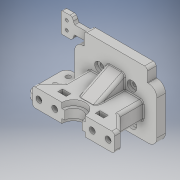
# Autodesk Inventor part: Froggie_DualFan_BLTouchMount01
Saved by Autodesk Inventor 2019.4 (Build 234330000, 330)
## iProperties
Created: 2019-11-18
Part Number: Froggie_DualFan_BLTouchMount01
Material: Generic
Document SubType Name: Modeling
Designer: frogm
Density: 1 g/cm^3
Appearance: Default
Author: frogm
Autodesk Inventor part; units mm, degrees
ref_plane "XZ Plane" through (0, 0, 0) normal (0, 1, 0) x (-1, 0, 0)
ref_plane "XY Plane" through (0, 0, 0) normal (0, 0, 1) x (1, 0, 0)
sketch "Base Sketch" plane through (0, 0, 0) normal (0, 0, 1) x (1, 0, 0)
  line L0 (0, 54) -> (0, -9) construction
  line L1 (-39.9, 0) -> (39.9, 0) construction
  line L2 (-28.5, 0) -> (28.5, 0)
  line L3 (-28.5, 0) -> (-28.5, 36)
  line L4 (-28.5, 36) -> (-22, 36)
  line L5 (-22, 36) -> (-22, 45)
  line L6 (-22, 45) -> (22, 45)
  line L7 (22, 45) -> (22, 36)
  line L8 (22, 36) -> (28.5, 36)
  line L9 (28.5, 36) -> (28.5, 0)
  point P0 (0, 0)
  point P1 (0, 0)
  dimension "d0" = 57
  dimension "d1" = 36
  dimension "d2" = 6.5
  dimension "d3" = 9
  dimension "d4" = 44
  dimension "d5" = 9
  dimension "d6" = 6.5
  dimension "d37" = 36
  constraints: 16 end point, 5 point on line, 4 perpendicular, 1 midpoint
  measures "d0" distance of L2.start L2.end
  measures "d1" distance of L2.start L3.end
  measures "d2" distance of L3.end L4.end
  measures "d3" distance of L4.end L5.end
  measures "d4" distance of L5.end L6.end
  measures "d5" distance of L6.end L7.end
  measures "d6" distance of L7.end L8.end
  measures "d37" distance of L8.end L2.end
extrude "Base Extrusion (6)" add sketch "Base Sketch" along normal blind 6
sketch "Base Holes Sketch" plane through (0, 0, 6) normal (0, 0, 1) x (1, 0, 0)
  line L0 (0, 0) -> (0, 44.9253) construction
  circle A0 centre (-11.25, 6.2) radius 1.5
  line L1 (-28.5, 0) -> (28.5, 0) projected
  circle A1 centre (11.25, 6.2) radius 1.5
  circle A2 centre (-11.25, 28.7) radius 1.5
  circle A3 centre (11.25, 28.7) radius 1.5
  circle A4 centre (-11.25, 6.2) radius 3.325
  circle A5 centre (11.25, 6.2) radius 3.325
  circle A6 centre (11.25, 28.7) radius 3.325
  circle A7 centre (-11.25, 28.7) radius 3.325
  dimension "d9" = 3
  dimension "d10" = 6.2
  dimension "d11" = 11.25
  dimension "d14" = 22.5
  dimension "d19" = 6.65
  dimension "d20" = 6.65
  dimension "d21" = 6.65
  dimension "d22" = 6.65
  constraints: 8 centre point, 4 coincident, 2 end point, 2 vertical, 1 symmetric about line, 5 other
  measures "d9" diameter of A0
  measures "d10" distance from line of L1 A0.centre
  measures "d11" distance from line of L0 A0.centre
  measures "d14" distance of A0.centre A2.centre
  measures "d19" diameter of A4
  measures "d20" diameter of A5
  measures "d21" diameter of A6
  measures "d22" diameter of A7
extrude "Base Screw Holes (Through)" cut sketch "Base Holes Sketch" against normal up to surface (6 mm away) contours A0 | A1 | A2 | A3
extrude "Counterbore Base Screws (2)" cut sketch "Base Holes Sketch" against normal blind 2
sketch "Heatsink Platform Sketch" plane through (0, 0, 6) normal (0, 0, 1) x (1, 0, 0)
  line L0 (28.5, 0) -> (28.5, 36) construction
  line L1 (-28.5, 36) -> (-28.5, 0) construction
  line L2 (-28.5, 17.45) -> (28.5, 17.45) construction
  circle A0 centre (-11.25, 28.7) radius 1.5 construction
  line L3 (-28.5, 23.8) -> (28.5, 23.8)
  line L4 (28.5, 23.8) -> (28.5, 11.1)
  line L5 (28.5, 11.1) -> (-28.5, 11.1)
  line L6 (-28.5, 11.1) -> (-28.5, 23.8)
  point P0 (0, 0)
  dimension "d27" = 11.25
  dimension "d28" = 12.7
  constraints: 10 end point, 5 point on line, 2 parallel, 2 perpendicular, 1 horizontal, 1 midpoint
  measures "d27" distance from line of A0.centre L2
  measures "d28" distance of L3.end L4.end
extrude "Heatsink Platform Extrusion (29.25)" add sketch "Heatsink Platform Sketch" along normal blind 29.25
sketch "Heatsink Platform Cutaway Sketch" plane through (-28.5, 23.8, 6) normal (0, 1, 0) x (1, 0, 0)
  line L0 (57, -29.25) -> (0, -29.25) construction
  line L1 (28.5, -29.25) -> (28.5, 0) construction
  line L2 (57, 0) -> (0, 0) construction
  line L3 (9.5, -16) -> (9.5, 0)
  line L4 (9.5, -16) -> (0, -25.35)
  line L5 (0, -25.35) -> (0, 0)
  line L6 (0, 0) -> (9.5, 0)
  line L7 (47.5, -16) -> (47.5, 0)
  line L8 (47.5, -16) -> (57, -25.35)
  line L9 (57, -25.35) -> (57, 0)
  line L10 (57, 0) -> (47.5, 0)
  point P0 (28.5, 6)
  dimension "d31" = 19
  dimension "d32" = 16
  dimension "d33" = 25.35
  constraints: 18 end point, 3 symmetric about line, 2 midpoint, 1 collinear, 1 perpendicular, 1 point on line
  measures "d31" distance from line of L1 L3.start
  measures "d32" distance from line of L2 L3.start
  measures "d33" distance from line of L2 L4.end
extrude "Heatsink Platform Cutaway Extrusion" cut sketch "Heatsink Platform Cutaway Sketch" against normal up to surface (12.7 mm away)
fillet "Heatsink Platform Trim Fillet (2)" radius 2 12 edges at (28.5, 23.8, 33.3) (23.75, 23.8, 26.675) (19, 23.8, 14) (19, 11.1, 14) (23.75, 11.1, 26.675) (28.5, 11.1, 33.3) (-19, 23.8, 14) (-23.75, 23.8, 26.675) (-28.5, 23.8, 33.3) (-28.5, 11.1, 33.3) (-23.75, 11.1, 26.675) (-19, 11.1, 14)
sketch "Heatsink Extrusion sketch" plane through (-17, 23.8, 6) normal (0, 1, 0) x (1, 0, 0)
  line L0 (43.5, -29.25) -> (-9.5, -29.25) projected
  arc A0 (23, -29.25) -> (11, -29.25) centre (17, -29.25) ccw
  arc A1 (25, -29.25) -> (9, -29.25) centre (17, -29.25) ccw
  line L1 (17, -29.25) -> (9, -29.25) construction
  line L2 (17, -29.25) -> (25, -29.25) construction
  line L3 (9, -29.25) -> (11, -29.25)
  line L4 (23, -29.25) -> (25, -29.25)
  line L5 (11, -29.25) -> (23, -29.25)
  point P0 (17, 6)
  dimension "d38" = 6
  dimension "d39" = 8
  dimension "d40" = 180
  constraints: 10 end point, 4 point on circle, 3 point on line, 2 centre point, 2 coincident, 2 collinear, 1 midpoint
  measures "d38" radius of A0
  measures "d39" radius of A1
  measures "d40" angle of L2 L1
extrude "Heatsink Center Extrusion (6)" cut sketch "Heatsink Extrusion sketch" against normal up to surface (12.7 mm away) contours L0 A0
extrude "Heastsink Top Outer Extrusion (3.7)" cut sketch "Heatsink Extrusion sketch" against normal blind 3.7 contours L0 A0 A1
sketch "Heatsink Bottom Extrusion Sketch" plane through (-17, 11.1, 6) normal (0, -1, 0) x (1, 0, 0)
  line L0 (11, 29.25) -> (9, 29.25) projected
  arc A0 (9, 29.25) -> (25, 29.25) centre (17, 29.25) ccw projected
  line L1 (25, 29.25) -> (23, 29.25) projected
  arc A1 (11, 29.25) -> (23, 29.25) centre (17, 29.25) ccw projected
  point P0 (17, -6)
extrude "Heatsink Bottom Outer Extrusion (3.0)" cut sketch "Heatsink Bottom Extrusion Sketch" against normal blind 3
ref_plane "Front Screw Hole Plane" through (0, 0, 35.25) normal (0, 0, 1) x (1, 0, 0)
sketch "Front Screw Hole Sketch" plane through (0, 0, 35.25) normal (0, 0, 1) x (1, 0, 0)
  line L0 (-8, 23.8) -> (-26.5, 23.8) construction
  line L1 (-8, 17.45) -> (-26.5, 17.45) construction
  line L2 (-28.5, 36) -> (-28.5, 0) construction
  line L3 (-28.5, 17.45) -> (28.5, 17.45) construction
  line L4 (-28.5, 17.45) -> (28.5, 17.45) construction
  line L5 (8, 11.1) -> (-8, 11.1) construction
  line L6 (0, 11.1) -> (0, 23.8) construction
  circle A0 centre (13, 17.45) radius 2.05
  circle A1 centre (-13, 17.45) radius 2.05
  circle A2 centre (24, 17.45) radius 2.05
  line L7 (28.5, 13.1) -> (28.5, 21.8) projected
  circle A3 centre (-24, 17.45) radius 2.05
  point P0 (0, 0)
  dimension "d48" = 6.35
  dimension "d49" = 57
  dimension "d50" = 0
  dimension "d51" = 4.1
  dimension "d52" = 13
  dimension "d53" = 4.1
  dimension "d54" = 4.5
  constraints: 8 end point, 4 centre point, 3 point on line, 2 collinear, 2 symmetric about line, 1 horizontal, 1 midpoint, 1 parallel, 1 vertical, 2 other
  measures "d48" distance between parallel lines of L0 L1
  measures "d49" distance of L3.start L3.end
  measures "d50" distance between parallel lines of L3 L4
  measures "d51" diameter of A0
  measures "d52" distance from line of L6 A0.centre
  measures "d53" diameter of A2
  measures "d54" distance from line of A2.centre L7
extrude "Heatsink Screw Hole Extrusion (14)" cut sketch "Front Screw Hole Sketch" against normal blind 14 contours A0 | A1
extrude "Hotend Cooling Fan Screw Holes Extrusion (To Next)" cut sketch "Front Screw Hole Sketch" against normal up to next contours A2 | A3
sketch "Nut-trap Sketch" plane through (-17, 23.8, 6) normal (0, 1, 0) x (1, 0, 0)
  arc A0 (25, -29.25) -> (9, -29.25) centre (17, -29.25) ccw construction
  line L0 (17, -21.25) -> (17, 0) construction
  line L1 (34, 0) -> (0, 0) construction
  line L2 (1.1, -24.25) -> (6.9, -24.25)
  line L3 (6.9, -24.25) -> (6.9, -21.05)
  line L4 (6.9, -21.05) -> (1.1, -21.05)
  line L5 (1.1, -21.05) -> (1.1, -24.25)
  line L6 (9, -29.25) -> (-9.5, -29.25) projected
  line L7 (32.9, -24.25) -> (27.1, -24.25)
  line L8 (27.1, -24.25) -> (27.1, -21.05)
  line L9 (27.1, -21.05) -> (32.9, -21.05)
  line L10 (32.9, -21.05) -> (32.9, -24.25)
  point P0 (17, 6)
  point P1 (4, -21.05)
  dimension "d59" = 5.8
  dimension "d60" = 3.2
  dimension "d61" = 5
  dimension "d62" = 13
  constraints: 18 end point, 4 symmetric about line, 2 midpoint, 2 parallel, 1 horizontal, 1 perpendicular, 1 point on circle, 1 vertical
  measures "d59" distance of L4.end L3.end
  measures "d60" distance of L3.end L2.end
  measures "d61" distance between parallel lines of L6 L2
  measures "d62" distance from line of L0 point (4, -21.05)
extrude "Nut-trap Extrusion (9.03)" cut sketch "Nut-trap Sketch" against normal blind 9.03
ref_plane "Cooling Fan Nut Sketch Plane" through (-17, 23.8, 22.8378) normal (0, 0, -1) x (-1, 0, 0)
sketch "Cooling Fan Nut Sketch" plane through (-17, 23.8, 22.8378) normal (0, 0, -1) x (-1, 0, 0)
  line L0 (3.8823, -6.3515) -> (5.4425, -9.0508)
  line L1 (5.4425, -9.0508) -> (8.5602, -9.0492)
  line L2 (8.5602, -9.0492) -> (10.1177, -6.3485)
  line L3 (10.1177, -6.3485) -> (8.5575, -3.6492)
  line L4 (8.5575, -3.6492) -> (5.4398, -3.6508)
  line L5 (5.4398, -3.6508) -> (3.8823, -6.3515)
  line L6 (7.0013, -9.05) -> (6.9987, -3.65) construction
  circle A0 centre (7, -6.35) radius 2.05 projected
  line L7 (-25, 0) -> (-9, 0) projected
  line L8 (-17, 0) -> (-17, -12.7) construction
  line L9 (-34, -12.7) -> (0, -12.7) projected
  line L10 (-37.8823, -6.3515) -> (-39.4425, -9.0508)
  line L11 (-39.4425, -9.0508) -> (-42.5602, -9.0492)
  line L12 (-42.5602, -9.0492) -> (-44.1177, -6.3485)
  line L13 (-44.1177, -6.3485) -> (-42.5575, -3.6492)
  line L14 (-42.5575, -3.6492) -> (-39.4398, -3.6508)
  line L15 (-39.4398, -3.6508) -> (-37.8823, -6.3515)
  point P0 (-17, -23.8)
  point P1 (7, -6.35)
  constraints: 28 end point, 6 symmetric about line, 5 midpoint
extrude "Cooling Fan Nut Extrusion (10.25)" cut sketch "Cooling Fan Nut Sketch" against normal blind 10.25 contours L5 L4 L3 L2 L1 L0 | A0 | L10 L11 L12 L13 L14 L15
ref_plane "Support Brace Plane" through (6.3, 0, 0) normal (1, 0, 0) x (0, 1, 0)
sketch "Top Support Brace Sketch" plane through (6.3, 0, 0) normal (1, 0, 0) x (0, 1, 0)
  line L0 (23.8, 6) -> (23.8, 26)
  line L1 (23.8, 6) -> (23.8, 22.8378) projected
  line L2 (23.8, 6) -> (33.8, 6)
  line L3 (33.8, 6) -> (23.8, 26)
  point P0 (0, 0)
  dimension "d68" = 20
  dimension "d69" = 10
  constraints: 6 end point, 1 collinear
  measures "d68" distance of L0.start L0.end
  measures "d69" distance of L0.start L2.end
extrude "Top Support Brace Extrusion (12.6)" add sketch "Top Support Brace Sketch" against normal blind 12.6
fillet "Support Base Trim Fillet (2)" radius 2 2 edges at (6.3, 28.8, 16) (-6.3, 28.8, 16)
fillet "Support Base Congruent Fillet (.6)" radius 0.6 10 edges at (5.7142, 23.8, 24.6901) (0, 23.8, 26) (-5.7142, 23.8, 24.6901) (-6.3, 23.8, 13.7639) (6.3, 23.8, 13.7639) (5.7142, 33.1451, 6) (0, 33.8, 6) (-5.7142, 33.1451, 6) (-6.3, 27.682, 6) (6.3, 27.682, 6)
fillet "Heatsink Platform Congruent Fillet (.6)" radius 0.6 11 edges at (11.95, 23.8, 6) (6.4757, 23.9757, 6.1757) (19, 17.45, 6) (18.4142, 11.6858, 6) (0, 11.1, 6) (-18.4142, 11.6858, 6) (-19, 17.45, 6) (-18.4142, 23.2142, 6) (-11.95, 23.8, 6) (-6.4757, 23.9757, 6.1757) (18.4142, 23.2142, 6)
ref_plane "Support Base Cross Section Plane" through (-17, 17.45, 22.8378) normal (0, 1, 0) x (1, 0, 0)
mirror "Support Base Mirror" about plane through (-17, 17.45, 22.8378) normal (0, 1, 0) of "Top Support Brace Extrusion (12.6)", "Support Base Trim Fillet (2)", "Support Base Congruent Fillet (.6)"
fillet "Base Large Fillet (6)" radius 6 4 edges at (28.5, 0, 3) (28.5, 36, 3) (-28.5, 36, 3) (-28.5, 0, 3)
fillet "Base Small Fillet (3)" radius 2 2 edges at (-22, 45, 3) (22, 45, 3)
ref_plane "BL Touch Platform Plane" through (-22.5, 6.75, 0) normal (0, -1, 0) x (1, 0, 0)
sketch "BL Touch Platform Sketch" plane through (-22.5, 6.75, 0) normal (0, -1, 0) x (1, 0, 0)
  line L0 (-6, 0) -> (-17.6, 0)
  line L1 (-17.6, 0) -> (-17.6, 27.5)
  line L2 (-17.6, 27.5) -> (-6, 27.5)
  line L3 (-6, 27.5) -> (-6, 0)
  point P0 (22.5, 0)
  dimension "d79" = 11.6
  dimension "d80" = 27.5
  constraints: 8 end point, 2 parallel, 1 horizontal, 1 perpendicular
  measures "d79" distance of L1.end L2.end
  measures "d80" distance of L0.end L1.end
extrude "BL Touch Platform Extrusion (4)" add sketch "BL Touch Platform Sketch" against normal blind 4
fillet "BL Touch Platform Trim Fillet (4.5)" radius 4.5 3 edges at (-40.1, 8.75, 0) (-40.1, 8.75, 27.5) (-28.5, 8.75, 27.5)
sketch "BL Touch Platform Holes Sketch" plane through (-22.5, 10.75, 0) normal (0, 1, 0) x (1, 0, 0)
  circle A0 centre (-11.765, -22.73) radius 1.6
  circle A1 centre (-11.765, -13.73) radius 1.6
  circle A2 centre (-11.765, -4.73) radius 1.6
  point P0 (22.5, 0)
  point P1 (22.5, -4)
  dimension "d86" = 3.2
  dimension "d91" = 3.2
  constraints: 3 centre point, 1 coincident
  measures "d86" diameter of A2
  measures "d91" diameter of A1
extrude "BL Touch Screw Holes Extrusion (Through)" cut sketch "BL Touch Platform Holes Sketch" against normal up to surface (4 mm away)
sketch "Endstop Holder Sketch" plane through (0, 0, 0) normal (0, 0, 1) x (1, 0, 0)
  line L0 (-31.8142, 34.5) -> (-31.8142, 32.7426) construction
  line L1 (-34.764, 32.3787) -> (-39.9355, 32.3787)
  arc A0 (-34.764, 32.3787) -> (-33.3497, 32.9645) centre (-34.764, 34.3787) ccw
  arc A1 (-40.9355, 33.3787) -> (-39.9355, 32.3787) centre (-39.9355, 33.3787) ccw
  arc A2 (-33.3497, 46.0355) -> (-34.764, 46.6213) centre (-34.764, 44.6213) ccw
  line L2 (-34.764, 46.6213) -> (-39.9355, 46.6213)
  arc A3 (-39.9355, 46.6213) -> (-40.9355, 45.6213) centre (-39.9355, 45.6213) ccw
  line L3 (-40.9355, 33.3787) -> (-40.9355, 45.6213)
  line L4 (-36.9355, 32.3787) -> (-36.9355, 46.6213) construction
  circle A4 centre (-36.9355, 36.5002) radius 1
  circle A5 centre (-36.9355, 42.5002) radius 1
  line L5 (-40.9355, 39.5) -> (-24.6363, 39.5) construction
  arc A6 (-32.2633, 44.3544) -> (-31.4, 42.5) centre (-28.7972, 44.8399) ccw
  arc A7 (-32.2633, 44.3544) -> (-33.3497, 46.0355) centre (-36.2903, 42.9436) ccw
  arc A8 (-31.4, 36.5) -> (-32.2633, 34.6456) centre (-28.7972, 34.1601) ccw
  arc A9 (-33.3497, 32.9645) -> (-32.2633, 34.6456) centre (-36.2903, 36.0564) ccw
  line L6 (-31.4, 42.5) -> (-22, 42.5)
  line L7 (-31.4, 36.5) -> (-22, 36.5)
  line L8 (-22, 36.5) -> (-22, 42.5)
  point P0 (-33.9355, 32.3787)
  point P1 (-40.9355, 32.3787)
  point P2 (-40.9355, 47.3787)
  point P3 (-33.9355, 47.3787)
  point P4 (-22, 36)
  dimension "d97" = 3
  dimension "d99" = 7
  dimension "d100" = 15
  dimension "d101" = 7
  dimension "d102" = 1
  dimension "d106" = 4
  dimension "d107" = 4.1215
  dimension "d108" = 6
  dimension "d109" = 4.1211
  dimension "d110" = 2
  dimension "d111" = 2
  dimension "d117" = 3.5
  dimension "d119" = 9.4
  constraints: 18 end point, 16 point on circle, 10 centre point, 4 point on line, 3 horizontal, 2 coincident, 2 tangent, 1 perpendicular
  measures "d97" distance of L0.start point (-33.936, 32.379)
  measures "d99" distance of point (-33.936, 32.379) point (-40.936, 32.379)
  measures "d100" distance of point (-40.936, 32.379) point (-40.936, 47.379)
  measures "d101" distance of point (-40.936, 47.379) point (-33.936, 47.379)
  measures "d102" radius of A1
  measures "d106" distance between parallel lines of L3 L4
  measures "d107" distance from line of L1 point (-36.936, 36.5)
  measures "d108" distance of point (-36.936, 36.5) point (-36.936, 42.5)
  measures "d109" distance from line of point (-36.936, 42.5) L2
  measures "d110" diameter of A4
  measures "d111" diameter of A5
  measures "d117" radius of A6
  measures "d119" distance of L6.start L6.end
extrude "Endstop Holder Extrusion (3)" add sketch "Endstop Holder Sketch" along normal blind 3 separate body
combine bodies "Combine2" operation type add bodies to combine 1 2
fillet "Combine Connecting Fillet (.6)" radius 0.6 2 edges at (-22, 36.5, 1.5) (-22, 42.5, 1.5)
body "Solid1"
